Autodesk Fusion 360 part; units mm, degrees
(part 2 of 7)
  line L506 (63.504, -56.2361) -> (63.4239, -56.2507)
  line L507 (63.4239, -56.2507) -> (63.3435, -56.2671)
  line L508 (63.3435, -56.2671) -> (63.3141, -56.4047)
  line L509 (63.3141, -56.4047) -> (63.2867, -56.5426)
  line L510 (63.2867, -56.5426) -> (63.2612, -56.681)
  line L511 (63.2612, -56.681) -> (63.3292, -56.7269)
  line L512 (63.3292, -56.7269) -> (63.3976, -56.7711)
  line L513 (63.3976, -56.7711) -> (63.4664, -56.8134)
  line L514 (63.4664, -56.8134) -> (63.5357, -56.8539)
  line L515 (63.5357, -56.8539) -> (63.6053, -56.8924)
  line L516 (63.6053, -56.8924) -> (63.6754, -56.9288)
  line L517 (63.6754, -56.9288) -> (63.7458, -56.9631)
  line L518 (63.7458, -56.9631) -> (63.8167, -56.9949)
  line L519 (63.8167, -56.9949) -> (63.888, -57.0242)
  line L520 (63.888, -57.0242) -> (63.9598, -57.0505)
  line L521 (63.9598, -57.0505) -> (64.0322, -57.0732)
  line L522 (64.0322, -57.0732) -> (64.1053, -57.0906)
  line L523 (64.1053, -57.0906) -> (64.512, -57.1506)
  line L524 (64.512, -57.1506) -> (64.484, -57.3575)
  line L525 (64.484, -57.3575) -> (64.461, -57.565)
  line L526 (64.461, -57.565) -> (64.443, -57.7729)
  line L527 (64.443, -57.7729) -> (64.4301, -57.9813)
  line L528 (64.4301, -57.9813) -> (64.0196, -57.9609)
  line L529 (64.0196, -57.9609) -> (63.9445, -57.9636)
  line L530 (63.9445, -57.9636) -> (63.8691, -57.9718)
  line L531 (63.8691, -57.9718) -> (63.7935, -57.9836)
  line L532 (63.7935, -57.9836) -> (63.7179, -57.9984)
  line L533 (63.7179, -57.9984) -> (63.6421, -58.0158)
  line L534 (63.6421, -58.0158) -> (63.5664, -58.0356)
  line L535 (63.5664, -58.0356) -> (63.4905, -58.0577)
  line L536 (63.4905, -58.0577) -> (63.4147, -58.0818)
  line L537 (63.4147, -58.0818) -> (63.3389, -58.108)
  line L538 (63.3389, -58.108) -> (63.2632, -58.1361)
  line L539 (63.2632, -58.1361) -> (63.1874, -58.1661)
  line L540 (63.1874, -58.1661) -> (63.1118, -58.1979)
  line L541 (63.1118, -58.1979) -> (63.1098, -58.3386)
  line L542 (63.1098, -58.3386) -> (63.1098, -58.4792)
  line L543 (63.1098, -58.4792) -> (63.1118, -58.6199)
  line L544 (63.1118, -58.6199) -> (63.1874, -58.6517)
  line L545 (63.1874, -58.6517) -> (63.2632, -58.6817)
  line L546 (63.2632, -58.6817) -> (63.3389, -58.7098)
  line L547 (63.3389, -58.7098) -> (63.4147, -58.7359)
  line L548 (63.4147, -58.7359) -> (63.4905, -58.7601)
  line L549 (63.4905, -58.7601) -> (63.5664, -58.7822)
  line L550 (63.5664, -58.7822) -> (63.6421, -58.802)
  line L551 (63.6421, -58.802) -> (63.7179, -58.8194)
  line L552 (63.7179, -58.8194) -> (63.7935, -58.8342)
  line L553 (63.7935, -58.8342) -> (63.8691, -58.846)
  line L554 (63.8691, -58.846) -> (63.9445, -58.8542)
  line L555 (63.9445, -58.8542) -> (64.0196, -58.8569)
  line L556 (64.0196, -58.8569) -> (64.4301, -58.8365)
  line L557 (64.4301, -58.8365) -> (64.443, -59.0449)
  line L558 (64.443, -59.0449) -> (64.461, -59.2528)
  line L559 (64.461, -59.2528) -> (64.484, -59.4603)
  line L560 (64.484, -59.4603) -> (64.512, -59.6672)
  line L561 (64.512, -59.6672) -> (64.1053, -59.7272)
  line L562 (64.1053, -59.7272) -> (64.0322, -59.7446)
  line L563 (64.0322, -59.7446) -> (63.9598, -59.7673)
  line L564 (63.9598, -59.7673) -> (63.888, -59.7936)
  line L565 (63.888, -59.7936) -> (63.8167, -59.8229)
  line L566 (63.8167, -59.8229) -> (63.7458, -59.8547)
  line L567 (63.7458, -59.8547) -> (63.6754, -59.889)
  line L568 (63.6754, -59.889) -> (63.6053, -59.9254)
  line L569 (63.6053, -59.9254) -> (63.5357, -59.9639)
  line L570 (63.5357, -59.9639) -> (63.4664, -60.0044)
  line L571 (63.4664, -60.0044) -> (63.3976, -60.0467)
  line L572 (63.3976, -60.0467) -> (63.3292, -60.0909)
  line L573 (63.3292, -60.0909) -> (63.2612, -60.1368)
  line L574 (63.2612, -60.1368) -> (63.2867, -60.2752)
  line L575 (63.2867, -60.2752) -> (63.3141, -60.4131)
  line L576 (63.3141, -60.4131) -> (63.3435, -60.5507)
  line L577 (63.3435, -60.5507) -> (63.4239, -60.5671)
  line L578 (63.4239, -60.5671) -> (63.504, -60.5817)
  line L579 (63.504, -60.5817) -> (63.5838, -60.5945)
  line L580 (63.5838, -60.5945) -> (63.6633, -60.6054)
  line L581 (63.6633, -60.6054) -> (63.7424, -60.6143)
  line L582 (63.7424, -60.6143) -> (63.821, -60.6212)
  line L583 (63.821, -60.6212) -> (63.8992, -60.6258)
  line L584 (63.8992, -60.6258) -> (63.9769, -60.6282)
  line L585 (63.9769, -60.6282) -> (64.054, -60.6279)
  line L586 (64.054, -60.6279) -> (64.1304, -60.6247)
  line L587 (64.1304, -60.6247) -> (64.2059, -60.618)
  line L588 (64.2059, -60.618) -> (64.2801, -60.6061)
  line L589 (64.2801, -60.6061) -> (64.6788, -60.5059)
  line L590 (64.6788, -60.5059) -> (64.7321, -60.7078)
  line L591 (64.7321, -60.7078) -> (64.7903, -60.9083)
  line L592 (64.7903, -60.9083) -> (64.8533, -61.1073)
  line L593 (64.8533, -61.1073) -> (64.9211, -61.3047)
  line L594 (64.9211, -61.3047) -> (64.534, -61.4429)
  line L595 (64.534, -61.4429) -> (64.4656, -61.4742)
  line L596 (64.4656, -61.4742) -> (64.3991, -61.5106)
  line L597 (64.3991, -61.5106) -> (64.3338, -61.5504)
  line L598 (64.3338, -61.5504) -> (64.2696, -61.593)
  line L599 (64.2696, -61.593) -> (64.2063, -61.6381)
  line L600 (64.2063, -61.6381) -> (64.1438, -61.6854)
  line L601 (64.1438, -61.6854) -> (64.0823, -61.7348)
  line L602 (64.0823, -61.7348) -> (64.0215, -61.7862)
  line L603 (64.0215, -61.7862) -> (63.9614, -61.8394)
  line L604 (63.9614, -61.8394) -> (63.9022, -61.8943)
  line L605 (63.9022, -61.8943) -> (63.8437, -61.951)
  line L606 (63.8437, -61.951) -> (63.786, -62.0093)
  line L607 (63.786, -62.0093) -> (63.8379, -62.14)
  line L608 (63.8379, -62.14) -> (63.8918, -62.27)
  line L609 (63.8918, -62.27) -> (63.9475, -62.3992)
  line L610 (63.9475, -62.3992) -> (64.0295, -62.3996)
  line L611 (64.0295, -62.3996) -> (64.111, -62.3983)
  line L612 (64.111, -62.3983) -> (64.1917, -62.3953)
  line L613 (64.1917, -62.3953) -> (64.2718, -62.3905)
  line L614 (64.2718, -62.3905) -> (64.3511, -62.3838)
  line L615 (64.3511, -62.3838) -> (64.4295, -62.3752)
  line L616 (64.4295, -62.3752) -> (64.5071, -62.3645)
  line L617 (64.5071, -62.3645) -> (64.5838, -62.3516)
  line L618 (64.5838, -62.3516) -> (64.6593, -62.3363)
  line L619 (64.6593, -62.3363) -> (64.7336, -62.3183)
  line L620 (64.7336, -62.3183) -> (64.8064, -62.297)
  line L621 (64.8064, -62.297) -> (64.8769, -62.2708)
  line L622 (64.8769, -62.2708) -> (65.2484, -62.0948)
  line L623 (65.2484, -62.0948) -> (65.34, -62.2823)
  line L624 (65.34, -62.2823) -> (65.4362, -62.4676)
  line L625 (65.4362, -62.4676) -> (65.5368, -62.6505)
  line L626 (65.5368, -62.6505) -> (65.6418, -62.8309)
  line L627 (65.6418, -62.8309) -> (65.2891, -63.042)
  line L628 (65.2891, -63.042) -> (65.2282, -63.086)
  line L629 (65.2282, -63.086) -> (65.17, -63.1347)
  line L630 (65.17, -63.1347) -> (65.1138, -63.1865)
  line L631 (65.1138, -63.1865) -> (65.0591, -63.2408)
  line L632 (65.0591, -63.2408) -> (65.0058, -63.2974)
  line L633 (65.0058, -63.2974) -> (64.9538, -63.356)
  line L634 (64.9538, -63.356) -> (64.903, -63.4164)
  line L635 (64.903, -63.4164) -> (64.8534, -63.4787)
  line L636 (64.8534, -63.4787) -> (64.8049, -63.5425)
  line L637 (64.8049, -63.5425) -> (64.7575, -63.608)
  line L638 (64.7575, -63.608) -> (64.7112, -63.675)
  line L639 (64.7112, -63.675) -> (64.666, -63.7435)
  line L640 (64.666, -63.7435) -> (64.7425, -63.8615)
  line L641 (64.7425, -63.8615) -> (64.8206, -63.9785)
  line L642 (64.8206, -63.9785) -> (64.9004, -64.0943)
  line L643 (64.9004, -64.0943) -> (64.981, -64.0787)
  line L644 (64.981, -64.0787) -> (65.0606, -64.0616)
  line L645 (65.0606, -64.0616) -> (65.1392, -64.0429)
  line L646 (65.1392, -64.0429) -> (65.2168, -64.0225)
  line L647 (65.2168, -64.0225) -> (65.2933, -64.0005)
  line L648 (65.2933, -64.0005) -> (65.3686, -63.9767)
  line L649 (65.3686, -63.9767) -> (65.4426, -63.9511)
  line L650 (65.4426, -63.9511) -> (65.5152, -63.9235)
  line L651 (65.5152, -63.9235) -> (65.5864, -63.8938)
  line L652 (65.5864, -63.8938) -> (65.6557, -63.8616)
  line L653 (65.6557, -63.8616) -> (65.723, -63.8265)
  line L654 (65.723, -63.8265) -> (65.787, -63.7871)
  line L655 (65.787, -63.7871) -> (66.117, -63.542)
  line L656 (66.117, -63.542) -> (66.2434, -63.7081)
  line L657 (66.2434, -63.7081) -> (66.3739, -63.871)
  line L658 (66.3739, -63.871) -> (66.5083, -64.0308)
  line L659 (66.5083, -64.0308) -> (66.6465, -64.1872)
  line L660 (66.6465, -64.1872) -> (66.3418, -64.4631)
  line L661 (66.3418, -64.4631) -> (66.2906, -64.5181)
  line L662 (66.2906, -64.5181) -> (66.243, -64.5772)
  line L663 (66.243, -64.5772) -> (66.1979, -64.639)
  line L664 (66.1979, -64.639) -> (66.1549, -64.7029)
  line L665 (66.1549, -64.7029) -> (66.1137, -64.7688)
  line L666 (66.1137, -64.7688) -> (66.0741, -64.8364)
  line L667 (66.0741, -64.8364) -> (66.0361, -64.9056)
  line L668 (66.0361, -64.9056) -> (65.9996, -64.9763)
  line L669 (65.9996, -64.9763) -> (65.9645, -65.0484)
  line L670 (65.9645, -65.0484) -> (65.9308, -65.1219)
  line L671 (65.9308, -65.1219) -> (65.8984, -65.1966)
  line L672 (65.8984, -65.1966) -> (65.8674, -65.2726)
  line L673 (65.8674, -65.2726) -> (65.9655, -65.3735)
  line L674 (65.9655, -65.3735) -> (66.0649, -65.473)
  line L675 (66.0649, -65.473) -> (66.1658, -65.571)
  line L676 (66.1658, -65.571) -> (66.2418, -65.54)
  line L677 (66.2418, -65.54) -> (66.3165, -65.5076)
  line L678 (66.3165, -65.5076) -> (66.39, -65.4739)
  line L679 (66.39, -65.4739) -> (66.4621, -65.4388)
  line L680 (66.4621, -65.4388) -> (66.5328, -65.4023)
  line L681 (66.5328, -65.4023) -> (66.602, -65.3643)
  line L682 (66.602, -65.3643) -> (66.6696, -65.3248)
  line L683 (66.6696, -65.3248) -> (66.7355, -65.2835)
  line L684 (66.7355, -65.2835) -> (66.7994, -65.2405)
  line L685 (66.7994, -65.2405) -> (66.8612, -65.1954)
  line L686 (66.8612, -65.1954) -> (66.9203, -65.1479)
  line L687 (66.9203, -65.1479) -> (66.9753, -65.0967)
  line L688 (66.9753, -65.0967) -> (67.2512, -64.7919)
  line L689 (67.2512, -64.7919) -> (67.4076, -64.9301)
  line L690 (67.4076, -64.9301) -> (67.5674, -65.0645)
  line L691 (67.5674, -65.0645) -> (67.7304, -65.195)
  line L692 (67.7304, -65.195) -> (67.8964, -65.3215)
  line L693 (67.8964, -65.3215) -> (67.6514, -65.6515)
  line L694 (67.6514, -65.6515) -> (67.6119, -65.7155)
  line L695 (67.6119, -65.7155) -> (67.5768, -65.7827)
  line L696 (67.5768, -65.7827) -> (67.5446, -65.8521)
  line L697 (67.5446, -65.8521) -> (67.5149, -65.9232)
  line L698 (67.5149, -65.9232) -> (67.4873, -65.9958)
  line L699 (67.4873, -65.9958) -> (67.4617, -66.0698)
  line L700 (67.4617, -66.0698) -> (67.4379, -66.1451)
  line L701 (67.4379, -66.1451) -> (67.4159, -66.2216)
  line L702 (67.4159, -66.2216) -> (67.3956, -66.2992)
  line L703 (67.3956, -66.2992) -> (67.3768, -66.3778)
  line L704 (67.3768, -66.3778) -> (67.3597, -66.4574)
  line L705 (67.3597, -66.4574) -> (67.3441, -66.538)
  line L706 (67.3441, -66.538) -> (67.4599, -66.6178)
  line L707 (67.4599, -66.6178) -> (67.5769, -66.6959)
  line L708 (67.5769, -66.6959) -> (67.695, -66.7724)
  line L709 (67.695, -66.7724) -> (67.7634, -66.7272)
  line L710 (67.7634, -66.7272) -> (67.8304, -66.6809)
  line L711 (67.8304, -66.6809) -> (67.8959, -66.6335)
  line L712 (67.8959, -66.6335) -> (67.9598, -66.585)
  line L713 (67.9598, -66.585) -> (68.022, -66.5354)
  line L714 (68.022, -66.5354) -> (68.0824, -66.4846)
  line L715 (68.0824, -66.4846) -> (68.141, -66.4326)
  line L716 (68.141, -66.4326) -> (68.1976, -66.3793)
  line L717 (68.1976, -66.3793) -> (68.2519, -66.3246)
  line L718 (68.2519, -66.3246) -> (68.3037, -66.2684)
  line L719 (68.3037, -66.2684) -> (68.3524, -66.2102)
  line L720 (68.3524, -66.2102) -> (68.3964, -66.1493)
  line L721 (68.3964, -66.1493) -> (68.6075, -65.7966)
  line L722 (68.6075, -65.7966) -> (68.7879, -65.9016)
  line L723 (68.7879, -65.9016) -> (68.9708, -66.0022)
  line L724 (68.9708, -66.0022) -> (69.1561, -66.0984)
  line L725 (69.1561, -66.0984) -> (69.3436, -66.19)
  line L726 (69.3436, -66.19) -> (69.1677, -66.5615)
  line L727 (69.1677, -66.5615) -> (69.1414, -66.632)
  line L728 (69.1414, -66.632) -> (69.1201, -66.7048)
  line L729 (69.1201, -66.7048) -> (69.1021, -66.7791)
  line L730 (69.1021, -66.7791) -> (69.0868, -66.8546)
  line L731 (69.0868, -66.8546) -> (69.0739, -66.9313)
  line L732 (69.0739, -66.9313) -> (69.0633, -67.0089)
  line L733 (69.0633, -67.0089) -> (69.0546, -67.0874)
  line L734 (69.0546, -67.0874) -> (69.0479, -67.1666)
  line L735 (69.0479, -67.1666) -> (69.0431, -67.2467)
  line L736 (69.0431, -67.2467) -> (69.0401, -67.3275)
  line L737 (69.0401, -67.3275) -> (69.0388, -67.4089)
  line L738 (69.0388, -67.4089) -> (69.0392, -67.491)
  line L739 (69.0392, -67.491) -> (69.1684, -67.5466)
  line L740 (69.1684, -67.5466) -> (69.2984, -67.6005)
  line L741 (69.2984, -67.6005) -> (69.4291, -67.6525)
  line L742 (69.4291, -67.6525) -> (69.4874, -67.5947)
  line L743 (69.4874, -67.5947) -> (69.5441, -67.5362)
  line L744 (69.5441, -67.5362) -> (69.5991, -67.477)
  line L745 (69.5991, -67.477) -> (69.6523, -67.417)
  line L746 (69.6523, -67.417) -> (69.7036, -67.3562)
  line L747 (69.7036, -67.3562) -> (69.753, -67.2946)
  line L748 (69.753, -67.2946) -> (69.8003, -67.2321)
  line L749 (69.8003, -67.2321) -> (69.8454, -67.1689)
  line L750 (69.8454, -67.1689) -> (69.888, -67.1046)
  line L751 (69.888, -67.1046) -> (69.9278, -67.0393)
  line L752 (69.9278, -67.0393) -> (69.9642, -66.9728)
  line L753 (69.9642, -66.9728) -> (69.9955, -66.9044)
  line L754 (69.9955, -66.9044) -> (70.1337, -66.5173)
  line L755 (70.1337, -66.5173) -> (70.3312, -66.5851)
  line L756 (70.3312, -66.5851) -> (70.5302, -66.6482)
  line L757 (70.5302, -66.6482) -> (70.7306, -66.7063)
  line L758 (70.7306, -66.7063) -> (70.9325, -66.7596)
  line L759 (70.9325, -66.7596) -> (70.8324, -67.1583)
  line L760 (70.8324, -67.1583) -> (70.8204, -67.2325)
  line L761 (70.8204, -67.2325) -> (70.8137, -67.3081)
  line L762 (70.8137, -67.3081) -> (70.8105, -67.3845)
  line L763 (70.8105, -67.3845) -> (70.8103, -67.4615)
  line L764 (70.8103, -67.4615) -> (70.8126, -67.5392)
  line L765 (70.8126, -67.5392) -> (70.8172, -67.6174)
  line L766 (70.8172, -67.6174) -> (70.8241, -67.6961)
  line L767 (70.8241, -67.6961) -> (70.833, -67.7751)
  line L768 (70.833, -67.7751) -> (70.8439, -67.8546)
  line L769 (70.8439, -67.8546) -> (70.8567, -67.9344)
  line L770 (70.8567, -67.9344) -> (70.8713, -68.0145)
  line L771 (70.8713, -68.0145) -> (70.8877, -68.0949)
  line L772 (70.8877, -68.0949) -> (71.0253, -68.1243)
  line L773 (71.0253, -68.1243) -> (71.1633, -68.1518)
  line L774 (71.1633, -68.1518) -> (71.3016, -68.1773)
  line L775 (71.3016, -68.1773) -> (71.3475, -68.1092)
  line L776 (71.3475, -68.1092) -> (71.3917, -68.0408)
  line L777 (71.3917, -68.0408) -> (71.4341, -67.972)
  line L778 (71.4341, -67.972) -> (71.4745, -67.9027)
  line L779 (71.4745, -67.9027) -> (71.513, -67.8331)
  line L780 (71.513, -67.8331) -> (71.5495, -67.7631)
  line L781 (71.5495, -67.7631) -> (71.5837, -67.6926)
  line L782 (71.5837, -67.6926) -> (71.6156, -67.6217)
  line L783 (71.6156, -67.6217) -> (71.6448, -67.5504)
  line L784 (71.6448, -67.5504) -> (71.6711, -67.4786)
  line L785 (71.6711, -67.4786) -> (71.6938, -67.4063)
  line L786 (71.6938, -67.4063) -> (71.7112, -67.3331)
  line L787 (71.7112, -67.3331) -> (71.7713, -66.9265)
  line L788 (71.7713, -66.9265) -> (71.9781, -66.9545)
  line L789 (71.9781, -66.9545) -> (72.1856, -66.9774)
  line L790 (72.1856, -66.9774) -> (72.3936, -66.9954)
  line L791 (72.3936, -66.9954) -> (72.6019, -67.0083)
  line L792 (72.6019, -67.0083) -> (72.5815, -67.4188)
  line L793 (72.5815, -67.4188) -> (72.5842, -67.494)
  line L794 (72.5842, -67.494) -> (72.5924, -67.5694)
  line L795 (72.5924, -67.5694) -> (72.6042, -67.6449)
  line L796 (72.6042, -67.6449) -> (72.619, -67.7206)
  line L797 (72.619, -67.7206) -> (72.6364, -67.7963)
  line L798 (72.6364, -67.7963) -> (72.6562, -67.8721)
  line L799 (72.6562, -67.8721) -> (72.6783, -67.9479)
  line L800 (72.6783, -67.9479) -> (72.7025, -68.0237)
  line L801 (72.7025, -68.0237) -> (72.7287, -68.0995)
  line L802 (72.7287, -68.0995) -> (72.7568, -68.1753)
  line L803 (72.7568, -68.1753) -> (72.7867, -68.251)
  line L804 (72.7867, -68.251) -> (72.8185, -68.3267)
  line L805 (72.8185, -68.3267) -> (72.9592, -68.3286)
  line L806 (72.9592, -68.3286) -> (73.0999, -68.3286)
  line L807 (73.0999, -68.3286) -> (73.2405, -68.3267)
  line L808 (73.2405, -68.3267) -> (73.2723, -68.251)
  line L809 (73.2723, -68.251) -> (73.3023, -68.1753)
  line L810 (73.3023, -68.1753) -> (73.3304, -68.0995)
  line L811 (73.3304, -68.0995) -> (73.3566, -68.0237)
  line L812 (73.3566, -68.0237) -> (73.3807, -67.9479)
  line L813 (73.3807, -67.9479) -> (73.4028, -67.8721)
  line L814 (73.4028, -67.8721) -> (73.4226, -67.7963)
  line L815 (73.4226, -67.7963) -> (73.4401, -67.7206)
  line L816 (73.4401, -67.7206) -> (73.4548, -67.6449)
  line L817 (73.4548, -67.6449) -> (73.4666, -67.5694)
  line L818 (73.4666, -67.5694) -> (73.4748, -67.494)
  line L819 (73.4748, -67.494) -> (73.4775, -67.4188)
  line L820 (73.4775, -67.4188) -> (73.4571, -67.0083)
  line L821 (73.4571, -67.0083) -> (73.6655, -66.9954)
  line L822 (73.6655, -66.9954) -> (73.8734, -66.9774)
  line L823 (73.8734, -66.9774) -> (74.0809, -66.9545)
  line L824 (74.0809, -66.9545) -> (74.2878, -66.9265)
  line L825 (74.2878, -66.9265) -> (74.3479, -67.3331)
  line L826 (74.3479, -67.3331) -> (74.3652, -67.4063)
  line L827 (74.3652, -67.4063) -> (74.3879, -67.4786)
  line L828 (74.3879, -67.4786) -> (74.4142, -67.5504)
  line L829 (74.4142, -67.5504) -> (74.4435, -67.6217)
  line L830 (74.4435, -67.6217) -> (74.4753, -67.6926)
  line L831 (74.4753, -67.6926) -> (74.5096, -67.7631)
  line L832 (74.5096, -67.7631) -> (74.546, -67.8331)
  line L833 (74.546, -67.8331) -> (74.5845, -67.9027)
  line L834 (74.5845, -67.9027) -> (74.625, -67.972)
  line L835 (74.625, -67.972) -> (74.6673, -68.0408)
  line L836 (74.6673, -68.0408) -> (74.7115, -68.1092)
  line L837 (74.7115, -68.1092) -> (74.7574, -68.1773)
  line L838 (74.7574, -68.1773) -> (74.8958, -68.1518)
  line L839 (74.8958, -68.1518) -> (75.0338, -68.1243)
  line L840 (75.0338, -68.1243) -> (75.1713, -68.0949)
  line L841 (75.1713, -68.0949) -> (75.1877, -68.0145)
  line L842 (75.1877, -68.0145) -> (75.2024, -67.9344)
  line L843 (75.2024, -67.9344) -> (75.2151, -67.8546)
  line L844 (75.2151, -67.8546) -> (75.226, -67.7751)
  line L845 (75.226, -67.7751) -> (75.235, -67.6961)
  line L846 (75.235, -67.6961) -> (75.2418, -67.6174)
  line L847 (75.2418, -67.6174) -> (75.2465, -67.5392)
  line L848 (75.2465, -67.5392) -> (75.2488, -67.4615)
  line L849 (75.2488, -67.4615) -> (75.2485, -67.3845)
  line L850 (75.2485, -67.3845) -> (75.2453, -67.3081)
  line L851 (75.2453, -67.3081) -> (75.2387, -67.2325)
  line L852 (75.2387, -67.2325) -> (75.2267, -67.1583)
  line L853 (75.2267, -67.1583) -> (75.1266, -66.7596)
  line L854 (75.1266, -66.7596) -> (75.3284, -66.7063)
  line L855 (75.3284, -66.7063) -> (75.5289, -66.6482)
  line L856 (75.5289, -66.6482) -> (75.7279, -66.5851)
  line L857 (75.7279, -66.5851) -> (75.9253, -66.5173)
  line L858 (75.9253, -66.5173) -> (76.0636, -66.9044)
  line L859 (76.0636, -66.9044) -> (76.0948, -66.9728)
  line L860 (76.0948, -66.9728) -> (76.1312, -67.0393)
  line L861 (76.1312, -67.0393) -> (76.171, -67.1046)
  line L862 (76.171, -67.1046) -> (76.2137, -67.1689)
  line L863 (76.2137, -67.1689) -> (76.2587, -67.2321)
  line L864 (76.2587, -67.2321) -> (76.306, -67.2946)
  line L865 (76.306, -67.2946) -> (76.3554, -67.3562)
  line L866 (76.3554, -67.3562) -> (76.4068, -67.417)
  line L867 (76.4068, -67.417) -> (76.46, -67.477)
  line L868 (76.46, -67.477) -> (76.515, -67.5362)
  line L869 (76.515, -67.5362) -> (76.5716, -67.5947)
  line L870 (76.5716, -67.5947) -> (76.6299, -67.6525)
  line L871 (76.6299, -67.6525) -> (76.7607, -67.6005)
  line L872 (76.7607, -67.6005) -> (76.8906, -67.5466)
  line L873 (76.8906, -67.5466) -> (77.0198, -67.491)
  line L874 (77.0198, -67.491) -> (77.0202, -67.4089)
  line L875 (77.0202, -67.4089) -> (77.0189, -67.3275)
  line L876 (77.0189, -67.3275) -> (77.0159, -67.2467)
  line L877 (77.0159, -67.2467) -> (77.0111, -67.1666)
  line L878 (77.0111, -67.1666) -> (77.0044, -67.0874)
  line L879 (77.0044, -67.0874) -> (76.9958, -67.0089)
  line L880 (76.9958, -67.0089) -> (76.9851, -66.9313)
  line L881 (76.9851, -66.9313) -> (76.9722, -66.8546)
  line L882 (76.9722, -66.8546) -> (76.9569, -66.7791)
  line L883 (76.9569, -66.7791) -> (76.9389, -66.7048)
  line L884 (76.9389, -66.7048) -> (76.9176, -66.632)
  line L885 (76.9176, -66.632) -> (76.8914, -66.5615)
  line L886 (76.8914, -66.5615) -> (76.7154, -66.19)
  line L887 (76.7154, -66.19) -> (76.903, -66.0984)
  line L888 (76.903, -66.0984) -> (77.0882, -66.0022)
  line L889 (77.0882, -66.0022) -> (77.2711, -65.9016)
  line L890 (77.2711, -65.9016) -> (77.4515, -65.7966)
  line L891 (77.4515, -65.7966) -> (77.6626, -66.1493)
  line L892 (77.6626, -66.1493) -> (77.7067, -66.2102)
  line L893 (77.7067, -66.2102) -> (77.7553, -66.2684)
  line L894 (77.7553, -66.2684) -> (77.8071, -66.3246)
  line L895 (77.8071, -66.3246) -> (77.8615, -66.3793)
  line L896 (77.8615, -66.3793) -> (77.918, -66.4326)
  line L897 (77.918, -66.4326) -> (77.9766, -66.4846)
  line L898 (77.9766, -66.4846) -> (78.0371, -66.5354)
  line L899 (78.0371, -66.5354) -> (78.0993, -66.585)
  line L900 (78.0993, -66.585) -> (78.1632, -66.6335)
  line L901 (78.1632, -66.6335) -> (78.2286, -66.6809)
  line L902 (78.2286, -66.6809) -> (78.2956, -66.7272)
  line L903 (78.2956, -66.7272) -> (78.3641, -66.7724)
  line L904 (78.3641, -66.7724) -> (78.4822, -66.6959)
  line L905 (78.4822, -66.6959) -> (78.5991, -66.6178)
  line L906 (78.5991, -66.6178) -> (78.715, -66.538)
  line L907 (78.715, -66.538) -> (78.6994, -66.4574)
  line L908 (78.6994, -66.4574) -> (78.6822, -66.3778)
  line L909 (78.6822, -66.3778) -> (78.6635, -66.2992)
  line L910 (78.6635, -66.2992) -> (78.6431, -66.2216)
  line L911 (78.6431, -66.2216) -> (78.6211, -66.1451)
  line L912 (78.6211, -66.1451) -> (78.5974, -66.0698)
  line L913 (78.5974, -66.0698) -> (78.5717, -65.9958)
  line L914 (78.5717, -65.9958) -> (78.5441, -65.9232)
  line L915 (78.5441, -65.9232) -> (78.5144, -65.8521)
  line L916 (78.5144, -65.8521) -> (78.4822, -65.7827)
  line L917 (78.4822, -65.7827) -> (78.4471, -65.7155)
  line L918 (78.4471, -65.7155) -> (78.4077, -65.6515)
  line L919 (78.4077, -65.6515) -> (78.1626, -65.3215)
  line L920 (78.1626, -65.3215) -> (78.3287, -65.195)
  line L921 (78.3287, -65.195) -> (78.4916, -65.0645)
  line L922 (78.4916, -65.0645) -> (78.6514, -64.9301)
  line L923 (78.6514, -64.9301) -> (78.8078, -64.7919)
  line L924 (78.8078, -64.7919) -> (79.0837, -65.0967)
  line L925 (79.0837, -65.0967) -> (79.1388, -65.1479)
  line L926 (79.1388, -65.1479) -> (79.1979, -65.1954)
  line L927 (79.1979, -65.1954) -> (79.2596, -65.2405)
  line L928 (79.2596, -65.2405) -> (79.3236, -65.2835)
  line L929 (79.3236, -65.2835) -> (79.3894, -65.3248)
  line L930 (79.3894, -65.3248) -> (79.457, -65.3643)
  line L931 (79.457, -65.3643) -> (79.5262, -65.4023)
  line L932 (79.5262, -65.4023) -> (79.5969, -65.4388)
  line L933 (79.5969, -65.4388) -> (79.6691, -65.4739)
  line L934 (79.6691, -65.4739) -> (79.7425, -65.5076)
  line L935 (79.7425, -65.5076) -> (79.8173, -65.54)
  line L936 (79.8173, -65.54) -> (79.8932, -65.571)
  line L937 (79.8932, -65.571) -> (79.9941, -65.473)
  line L938 (79.9941, -65.473) -> (80.0936, -65.3735)
  line L939 (80.0936, -65.3735) -> (80.1916, -65.2726)
  line L940 (80.1916, -65.2726) -> (80.1606, -65.1966)
  line L941 (80.1606, -65.1966) -> (80.1283, -65.1219)
  line L942 (80.1283, -65.1219) -> (80.0945, -65.0484)
  line L943 (80.0945, -65.0484) -> (80.0595, -64.9763)
  line L944 (80.0595, -64.9763) -> (80.0229, -64.9056)
  line L945 (80.0229, -64.9056) -> (79.9849, -64.8364)
  line L946 (79.9849, -64.8364) -> (79.9454, -64.7688)
  line L947 (79.9454, -64.7688) -> (79.9041, -64.7029)
  line L948 (79.9041, -64.7029) -> (79.8611, -64.639)
  line L949 (79.8611, -64.639) -> (79.816, -64.5772)
  line L950 (79.816, -64.5772) -> (79.7685, -64.5181)
  line L951 (79.7685, -64.5181) -> (79.7173, -64.4631)
  line L952 (79.7173, -64.4631) -> (79.4126, -64.1872)
  line L953 (79.4126, -64.1872) -> (79.5508, -64.0308)
  line L954 (79.5508, -64.0308) -> (79.6851, -63.871)
  line L955 (79.6851, -63.871) -> (79.8156, -63.7081)
  line L956 (79.8156, -63.7081) -> (79.9421, -63.542)
  line L957 (79.9421, -63.542) -> (80.2721, -63.7871)
  line L958 (80.2721, -63.7871) -> (80.3361, -63.8265)
  line L959 (80.3361, -63.8265) -> (80.4033, -63.8616)
  line L960 (80.4033, -63.8616) -> (80.4727, -63.8938)
  line L961 (80.4727, -63.8938) -> (80.5438, -63.9235)
  line L962 (80.5438, -63.9235) -> (80.6164, -63.9511)
  line L963 (80.6164, -63.9511) -> (80.6905, -63.9767)
  line L964 (80.6905, -63.9767) -> (80.7658, -64.0005)
  line L965 (80.7658, -64.0005) -> (80.8422, -64.0225)
  line L966 (80.8422, -64.0225) -> (80.9198, -64.0429)
  line L967 (80.9198, -64.0429) -> (80.9984, -64.0616)
  line L968 (80.9984, -64.0616) -> (81.078, -64.0787)
  line L969 (81.078, -64.0787) -> (81.1586, -64.0943)
  line L970 (81.1586, -64.0943) -> (81.2384, -63.9785)
  line L971 (81.2384, -63.9785) -> (81.3166, -63.8615)
  line L972 (81.3166, -63.8615) -> (81.3931, -63.7435)
  line L973 (81.3931, -63.7435) -> (81.3478, -63.675)
  line L974 (81.3478, -63.675) -> (81.3015, -63.608)
  line L975 (81.3015, -63.608) -> (81.2541, -63.5425)
  line L976 (81.2541, -63.5425) -> (81.2056, -63.4787)
  line L977 (81.2056, -63.4787) -> (81.156, -63.4164)
  line L978 (81.156, -63.4164) -> (81.1052, -63.356)
  line L979 (81.1052, -63.356) -> (81.0532, -63.2974)
  line L980 (81.0532, -63.2974) -> (81, -63.2408)
  line L981 (81, -63.2408) -> (80.9453, -63.1865)
  line L982 (80.9453, -63.1865) -> (80.889, -63.1347)
  line L983 (80.889, -63.1347) -> (80.8309, -63.086)
  line L984 (80.8309, -63.086) -> (80.7699, -63.042)
  line L985 (80.7699, -63.042) -> (80.4172, -62.8309)
  line L986 (80.4172, -62.8309) -> (80.5222, -62.6505)
  line L987 (80.5222, -62.6505) -> (80.6229, -62.4676)
  line L988 (80.6229, -62.4676) -> (80.719, -62.2823)
  line L989 (80.719, -62.2823) -> (80.8107, -62.0948)
  line L990 (80.8107, -62.0948) -> (81.1821, -62.2708)
  line L991 (81.1821, -62.2708) -> (81.2526, -62.297)
  line L992 (81.2526, -62.297) -> (81.3254, -62.3183)
  line L993 (81.3254, -62.3183) -> (81.3997, -62.3363)
  line L994 (81.3997, -62.3363) -> (81.4753, -62.3516)
  line L995 (81.4753, -62.3516) -> (81.5519, -62.3645)
  line L996 (81.5519, -62.3645) -> (81.6295, -62.3752)
  line L997 (81.6295, -62.3752) -> (81.708, -62.3838)
  line L998 (81.708, -62.3838) -> (81.7873, -62.3905)
  line L999 (81.7873, -62.3905) -> (81.8673, -62.3953)
  line L1000 (81.8673, -62.3953) -> (81.9481, -62.3983)
  line L1001 (81.9481, -62.3983) -> (82.0295, -62.3996)
  line L1002 (82.0295, -62.3996) -> (82.1116, -62.3992)
  line L1003 (82.1116, -62.3992) -> (82.1673, -62.27)
  line L1004 (82.1673, -62.27) -> (82.2211, -62.14)
  line L1005 (82.2211, -62.14) -> (82.2731, -62.0093)
  line L1006 (82.2731, -62.0093) -> (82.2153, -61.951)
  line L1007 (82.2153, -61.951) -> (82.1568, -61.8943)
  line L1008 (82.1568, -61.8943) -> (82.0976, -61.8394)
  line L1009 (82.0976, -61.8394) -> (82.0376, -61.7862)
  line L1010 (82.0376, -61.7862) -> (81.9768, -61.7348)
  line L1011 (81.9768, -61.7348) -> (81.9152, -61.6854)
  line L1012 (81.9152, -61.6854) -> (81.8528, -61.6381)
  line L1013 (81.8528, -61.6381) -> (81.7895, -61.593)
  line L1014 (81.7895, -61.593) -> (81.7252, -61.5504)
  line L1015 (81.7252, -61.5504) -> (81.6599, -61.5106)
  line L1016 (81.6599, -61.5106) -> (81.5934, -61.4742)
  line L1017 (81.5934, -61.4742) -> (81.525, -61.4429)
  line L1018 (81.525, -61.4429) -> (81.1379, -61.3047)
  line L1019 (81.1379, -61.3047) -> (81.2058, -61.1073)
  line L1020 (81.2058, -61.1073) -> (81.2688, -60.9083)
  line L1021 (81.2688, -60.9083) -> (81.3269, -60.7078)
  line L1022 (81.3269, -60.7078) -> (81.3802, -60.5059)
  line L1023 (81.3802, -60.5059) -> (81.7789, -60.6061)
  line L1024 (81.7789, -60.6061) -> (81.8531, -60.618)
  line L1025 (81.8531, -60.618) -> (81.9287, -60.6247)
  line L1026 (81.9287, -60.6247) -> (82.0051, -60.6279)
  line L1027 (82.0051, -60.6279) -> (82.0822, -60.6282)
  line L1028 (82.0822, -60.6282) -> (82.1598, -60.6258)
  line L1029 (82.1598, -60.6258) -> (82.238, -60.6212)
  line L1030 (82.238, -60.6212) -> (82.3167, -60.6143)
  line L1031 (82.3167, -60.6143) -> (82.3958, -60.6054)
  line L1032 (82.3958, -60.6054) -> (82.4752, -60.5945)
  line L1033 (82.4752, -60.5945) -> (82.555, -60.5817)
  line L1034 (82.555, -60.5817) -> (82.6351, -60.5671)
  line L1035 (82.6351, -60.5671) -> (82.7155, -60.5507)
  line L1036 (82.7155, -60.5507) -> (82.7449, -60.4131)
  line L1037 (82.7449, -60.4131) -> (82.7724, -60.2752)
  line L1038 (82.7724, -60.2752) -> (82.7979, -60.1368)
  line L1039 (82.7979, -60.1368) -> (82.7299, -60.0909)
  line L1040 (82.7299, -60.0909) -> (82.6614, -60.0467)
  line L1041 (82.6614, -60.0467) -> (82.5926, -60.0044)
  line L1042 (82.5926, -60.0044) -> (82.5234, -59.9639)
  line L1043 (82.5234, -59.9639) -> (82.4537, -59.9254)
  line L1044 (82.4537, -59.9254) -> (82.3837, -59.889)
  line L1045 (82.3837, -59.889) -> (82.3132, -59.8547)
  line L1046 (82.3132, -59.8547) -> (82.2423, -59.8229)
  line L1047 (82.2423, -59.8229) -> (82.171, -59.7936)
  line L1048 (82.171, -59.7936) -> (82.0992, -59.7673)
  line L1049 (82.0992, -59.7673) -> (82.0269, -59.7446)
  line L1050 (82.0269, -59.7446) -> (81.9537, -59.7272)
  line L1051 (81.9537, -59.7272) -> (81.5471, -59.6672)
  line L1052 (81.5471, -59.6672) -> (81.5751, -59.4603)
  line L1053 (81.5751, -59.4603) -> (81.5981, -59.2528)
  line L1054 (81.5981, -59.2528) -> (81.616, -59.0449)
  line L1055 (81.616, -59.0449) -> (81.6289, -58.8365)
  circle A0 centre (73.0295, -58.4089) radius 2.2
extrude "Extrude1'" add sketch "Sketch1 (2)" along normal blind 2 separate body makes body 2 in component "CT idler 1"
ref_plane "WorkPlane2" through (0, 0, 39) normal (0, 0, 1) x (1, 0, 0) in component "CT idler 1"
sketch "Sketch2" plane through (0, 0, 39) normal (0, 0, 1) x (1, 0, 0) in component "CT idler 1"
  line L0 (76.0819, -58.8895) -> (76.3712, -58.9351)
  line L1 (76.3712, -58.9351) -> (76.4518, -58.9359)
  line L2 (76.4518, -58.9359) -> (76.5339, -58.9268)
  line L3 (76.5339, -58.9268) -> (76.6168, -58.9107)
  line L4 (76.6168, -58.9107) -> (76.7002, -58.8887)
  line L5 (76.7002, -58.8887) -> (76.7841, -58.8612)
  line L6 (76.7841, -58.8612) -> (76.8681, -58.8287)
  line L7 (76.8681, -58.8287) -> (76.9521, -58.7913)
  line L8 (76.9521, -58.7913) -> (77.036, -58.7493)
  line L9 (77.036, -58.7493) -> (77.1197, -58.7028)
  line L10 (77.1197, -58.7028) -> (77.2029, -58.6518)
  line L11 (77.2029, -58.6518) -> (77.2856, -58.5964)
  line L12 (77.2856, -58.5964) -> (77.3676, -58.5368)
  line L13 (77.3676, -58.5368) -> (77.3693, -58.4515)
  line L14 (77.3693, -58.4515) -> (77.3693, -58.3662)
  line L15 (77.3693, -58.3662) -> (77.3676, -58.281)
  line L16 (77.3676, -58.281) -> (77.2856, -58.2214)
  line L17 (77.2856, -58.2214) -> (77.2029, -58.166)
  line L18 (77.2029, -58.166) -> (77.1197, -58.115)
  line L19 (77.1197, -58.115) -> (77.036, -58.0685)
  line L20 (77.036, -58.0685) -> (76.9521, -58.0265)
  line L21 (76.9521, -58.0265) -> (76.8681, -57.9891)
  line L22 (76.8681, -57.9891) -> (76.7841, -57.9566)
  line L23 (76.7841, -57.9566) -> (76.7002, -57.9291)
  line L24 (76.7002, -57.9291) -> (76.6168, -57.9071)
  line L25 (76.6168, -57.9071) -> (76.5339, -57.891)
  line L26 (76.5339, -57.891) -> (76.4518, -57.8819)
  line L27 (76.4518, -57.8819) -> (76.3712, -57.8827)
  line L28 (76.3712, -57.8827) -> (76.0819, -57.9283)
  line L29 (76.0819, -57.9283) -> (76.0523, -57.7678)
  line L30 (76.0523, -57.7678) -> (76.0142, -57.6091)
  line L31 (76.0142, -57.6091) -> (75.9679, -57.4527)
  line L32 (75.9679, -57.4527) -> (75.9133, -57.2989)
  line L33 (75.9133, -57.2989) -> (76.1866, -57.1937)
  line L34 (76.1866, -57.1937) -> (76.2568, -57.1542)
  line L35 (76.2568, -57.1542) -> (76.3233, -57.1052)
  line L36 (76.3233, -57.1052) -> (76.3871, -57.0499)
  line L37 (76.3871, -57.0499) -> (76.4483, -56.989)
  line L38 (76.4483, -56.989) -> (76.5072, -56.9233)
  line L39 (76.5072, -56.9233) -> (76.5637, -56.8532)
  line L40 (76.5637, -56.8532) -> (76.6178, -56.7788)
  line L41 (76.6178, -56.7788) -> (76.6695, -56.7005)
  line L42 (76.6695, -56.7005) -> (76.7187, -56.6183)
  line L43 (76.7187, -56.6183) -> (76.7652, -56.5325)
  line L44 (76.7652, -56.5325) -> (76.8092, -56.4433)
  line L45 (76.8092, -56.4433) -> (76.8504, -56.3506)
  line L46 (76.8504, -56.3506) -> (76.8092, -56.2759)
  line L47 (76.8092, -56.2759) -> (76.7666, -56.2021)
  line L48 (76.7666, -56.2021) -> (76.7225, -56.129)
  line L49 (76.7225, -56.129) -> (76.6217, -56.1184)
  line L50 (76.6217, -56.1184) -> (76.5224, -56.1119)
  line L51 (76.5224, -56.1119) -> (76.4248, -56.1093)
  line L52 (76.4248, -56.1093) -> (76.3291, -56.1108)
  line L53 (76.3291, -56.1108) -> (76.2354, -56.1164)
  line L54 (76.2354, -56.1164) -> (76.1439, -56.1261)
  line L55 (76.1439, -56.1261) -> (76.0549, -56.1399)
  line L56 (76.0549, -56.1399) -> (75.9686, -56.1581)
  line L57 (75.9686, -56.1581) -> (75.8853, -56.1807)
  line L58 (75.8853, -56.1807) -> (75.8054, -56.2082)
  line L59 (75.8054, -56.2082) -> (75.7298, -56.2413)
  line L60 (75.7298, -56.2413) -> (75.6604, -56.2823)
  line L61 (75.6604, -56.2823) -> (75.4327, -56.4665)
  line L62 (75.4327, -56.4665) -> (75.3268, -56.3423)
  line L63 (75.3268, -56.3423) -> (75.2145, -56.2239)
  line L64 (75.2145, -56.2239) -> (75.0961, -56.1117)
  line L65 (75.0961, -56.1117) -> (74.972, -56.0058)
  line L66 (74.972, -56.0058) -> (75.1561, -55.778)
  line L67 (75.1561, -55.778) -> (75.1971, -55.7086)
  line L68 (75.1971, -55.7086) -> (75.2302, -55.633)
  line L69 (75.2302, -55.633) -> (75.2577, -55.5532)
  line L70 (75.2577, -55.5532) -> (75.2804, -55.4699)
  line L71 (75.2804, -55.4699) -> (75.2985, -55.3835)
  line L72 (75.2985, -55.3835) -> (75.3124, -55.2945)
  line L73 (75.3124, -55.2945) -> (75.322, -55.203)
  line L74 (75.322, -55.203) -> (75.3276, -55.1094)
  line L75 (75.3276, -55.1094) -> (75.3291, -55.0136)
  line L76 (75.3291, -55.0136) -> (75.3266, -54.916)
  line L77 (75.3266, -54.916) -> (75.32, -54.8168)
  line L78 (75.32, -54.8168) -> (75.3094, -54.7159)
  line L79 (75.3094, -54.7159) -> (75.2364, -54.6719)
  line L80 (75.2364, -54.6719) -> (75.1625, -54.6292)
  line L81 (75.1625, -54.6292) -> (75.0878, -54.588)
  line L82 (75.0878, -54.588) -> (74.9952, -54.6292)
  line L83 (74.9952, -54.6292) -> (74.9059, -54.6732)
  line L84 (74.9059, -54.6732) -> (74.8201, -54.7198)
  line L85 (74.8201, -54.7198) -> (74.738, -54.7689)
  line L86 (74.738, -54.7689) -> (74.6596, -54.8206)
  line L87 (74.6596, -54.8206) -> (74.5852, -54.8747)
  line L88 (74.5852, -54.8747) -> (74.5151, -54.9312)
  line L89 (74.5151, -54.9312) -> (74.4494, -54.9901)
  line L90 (74.4494, -54.9901) -> (74.3886, -55.0514)
  line L91 (74.3886, -55.0514) -> (74.3332, -55.1151)
  line L92 (74.3332, -55.1151) -> (74.2842, -55.1816)
  line L93 (74.2842, -55.1816) -> (74.2447, -55.2518)
  line L94 (74.2447, -55.2518) -> (74.1395, -55.5251)
  line L95 (74.1395, -55.5251) -> (73.9857, -55.4706)
  line L96 (73.9857, -55.4706) -> (73.8293, -55.4242)
  line L97 (73.8293, -55.4242) -> (73.6706, -55.3861)
  line L98 (73.6706, -55.3861) -> (73.5102, -55.3565)
  line L99 (73.5102, -55.3565) -> (73.5557, -55.0672)
  line L100 (73.5557, -55.0672) -> (73.5566, -54.9866)
  line L101 (73.5566, -54.9866) -> (73.5474, -54.9046)
  line L102 (73.5474, -54.9046) -> (73.5313, -54.8217)
  line L103 (73.5313, -54.8217) -> (73.5093, -54.7382)
  line L104 (73.5093, -54.7382) -> (73.4818, -54.6544)
  line L105 (73.4818, -54.6544) -> (73.4493, -54.5703)
  line L106 (73.4493, -54.5703) -> (73.412, -54.4863)
  line L107 (73.412, -54.4863) -> (73.3699, -54.4024)
  line L108 (73.3699, -54.4024) -> (73.3234, -54.3187)
  line L109 (73.3234, -54.3187) -> (73.2724, -54.2355)
  line L110 (73.2724, -54.2355) -> (73.2171, -54.1528)
  line L111 (73.2171, -54.1528) -> (73.1575, -54.0708)
  line L112 (73.1575, -54.0708) -> (73.0722, -54.0691)
  line L113 (73.0722, -54.0691) -> (72.9869, -54.0691)
  line L114 (72.9869, -54.0691) -> (72.9016, -54.0708)
  line L115 (72.9016, -54.0708) -> (72.842, -54.1528)
  line L116 (72.842, -54.1528) -> (72.7866, -54.2355)
  line L117 (72.7866, -54.2355) -> (72.7357, -54.3187)
  line L118 (72.7357, -54.3187) -> (72.6891, -54.4024)
  line L119 (72.6891, -54.4024) -> (72.6471, -54.4863)
  line L120 (72.6471, -54.4863) -> (72.6097, -54.5703)
  line L121 (72.6097, -54.5703) -> (72.5772, -54.6544)
  line L122 (72.5772, -54.6544) -> (72.5498, -54.7382)
  line L123 (72.5498, -54.7382) -> (72.5277, -54.8217)
  line L124 (72.5277, -54.8217) -> (72.5116, -54.9046)
  line L125 (72.5116, -54.9046) -> (72.5025, -54.9866)
  line L126 (72.5025, -54.9866) -> (72.5033, -55.0672)
  line L127 (72.5033, -55.0672) -> (72.5489, -55.3565)
  line L128 (72.5489, -55.3565) -> (72.3884, -55.3861)
  line L129 (72.3884, -55.3861) -> (72.2298, -55.4242)
  line L130 (72.2298, -55.4242) -> (72.0733, -55.4706)
  line L131 (72.0733, -55.4706) -> (71.9196, -55.5251)
  line L132 (71.9196, -55.5251) -> (71.8144, -55.2518)
  line L133 (71.8144, -55.2518) -> (71.7748, -55.1816)
  line L134 (71.7748, -55.1816) -> (71.7259, -55.1151)
  line L135 (71.7259, -55.1151) -> (71.6705, -55.0514)
  line L136 (71.6705, -55.0514) -> (71.6097, -54.9901)
  line L137 (71.6097, -54.9901) -> (71.544, -54.9312)
  line L138 (71.544, -54.9312) -> (71.4738, -54.8747)
  line L139 (71.4738, -54.8747) -> (71.3994, -54.8206)
  line L140 (71.3994, -54.8206) -> (71.3211, -54.7689)
  line L141 (71.3211, -54.7689) -> (71.2389, -54.7198)
  line L142 (71.2389, -54.7198) -> (71.1531, -54.6732)
  line L143 (71.1531, -54.6732) -> (71.0639, -54.6292)
  line L144 (71.0639, -54.6292) -> (70.9713, -54.588)
  line L145 (70.9713, -54.588) -> (70.8966, -54.6292)
  line L146 (70.8966, -54.6292) -> (70.8227, -54.6719)
  line L147 (70.8227, -54.6719) -> (70.7497, -54.7159)
  line L148 (70.7497, -54.7159) -> (70.7391, -54.8168)
  line L149 (70.7391, -54.8168) -> (70.7325, -54.916)
  line L150 (70.7325, -54.916) -> (70.7299, -55.0136)
  line L151 (70.7299, -55.0136) -> (70.7314, -55.1094)
  line L152 (70.7314, -55.1094) -> (70.737, -55.203)
  line L153 (70.737, -55.203) -> (70.7467, -55.2945)
  line L154 (70.7467, -55.2945) -> (70.7605, -55.3835)
  line L155 (70.7605, -55.3835) -> (70.7787, -55.4699)
  line L156 (70.7787, -55.4699) -> (70.8013, -55.5532)
  line L157 (70.8013, -55.5532) -> (70.8288, -55.633)
  line L158 (70.8288, -55.633) -> (70.8619, -55.7086)
  line L159 (70.8619, -55.7086) -> (70.903, -55.778)
  line L160 (70.903, -55.778) -> (71.0871, -56.0058)
  line L161 (71.0871, -56.0058) -> (70.9629, -56.1117)
  line L162 (70.9629, -56.1117) -> (70.8446, -56.2239)
  line L163 (70.8446, -56.2239) -> (70.7323, -56.3423)
  line L164 (70.7323, -56.3423) -> (70.6264, -56.4665)
  line L165 (70.6264, -56.4665) -> (70.3986, -56.2823)
  line L166 (70.3986, -56.2823) -> (70.3292, -56.2413)
  line L167 (70.3292, -56.2413) -> (70.2536, -56.2082)
  line L168 (70.2536, -56.2082) -> (70.1738, -56.1807)
  line L169 (70.1738, -56.1807) -> (70.0905, -56.1581)
  line L170 (70.0905, -56.1581) -> (70.0042, -56.1399)
  line L171 (70.0042, -56.1399) -> (69.9151, -56.1261)
  line L172 (69.9151, -56.1261) -> (69.8237, -56.1164)
  line L173 (69.8237, -56.1164) -> (69.73, -56.1108)
  line L174 (69.73, -56.1108) -> (69.6343, -56.1093)
  line L175 (69.6343, -56.1093) -> (69.5367, -56.1119)
  line L176 (69.5367, -56.1119) -> (69.4374, -56.1184)
  line L177 (69.4374, -56.1184) -> (69.3366, -56.129)
  line L178 (69.3366, -56.129) -> (69.2925, -56.2021)
  line L179 (69.2925, -56.2021) -> (69.2498, -56.2759)
  line L180 (69.2498, -56.2759) -> (69.2086, -56.3506)
  line L181 (69.2086, -56.3506) -> (69.2499, -56.4433)
  line L182 (69.2499, -56.4433) -> (69.2938, -56.5325)
  line L183 (69.2938, -56.5325) -> (69.3404, -56.6183)
  line L184 (69.3404, -56.6183) -> (69.3896, -56.7005)
  line L185 (69.3896, -56.7005) -> (69.4412, -56.7788)
  line L186 (69.4412, -56.7788) -> (69.4953, -56.8532)
  line L187 (69.4953, -56.8532) -> (69.5518, -56.9233)
  line L188 (69.5518, -56.9233) -> (69.6107, -56.989)
  line L189 (69.6107, -56.989) -> (69.672, -57.0499)
  line L190 (69.672, -57.0499) -> (69.7357, -57.1052)
  line L191 (69.7357, -57.1052) -> (69.8022, -57.1542)
  line L192 (69.8022, -57.1542) -> (69.8724, -57.1937)
  line L193 (69.8724, -57.1937) -> (70.1458, -57.2989)
  line L194 (70.1458, -57.2989) -> (70.0912, -57.4527)
  line L195 (70.0912, -57.4527) -> (70.0448, -57.6091)
  line L196 (70.0448, -57.6091) -> (70.0068, -57.7678)
  line L197 (70.0068, -57.7678) -> (69.9771, -57.9283)
  line L198 (69.9771, -57.9283) -> (69.6878, -57.8827)
  line L199 (69.6878, -57.8827) -> (69.6072, -57.8819)
  line L200 (69.6072, -57.8819) -> (69.5252, -57.891)
  line L201 (69.5252, -57.891) -> (69.4423, -57.9071)
  line L202 (69.4423, -57.9071) -> (69.3588, -57.9291)
  line L203 (69.3588, -57.9291) -> (69.275, -57.9566)
  line L204 (69.275, -57.9566) -> (69.191, -57.9891)
  line L205 (69.191, -57.9891) -> (69.1069, -58.0265)
  line L206 (69.1069, -58.0265) -> (69.023, -58.0685)
  line L207 (69.023, -58.0685) -> (68.9393, -58.115)
  line L208 (68.9393, -58.115) -> (68.8561, -58.166)
  line L209 (68.8561, -58.166) -> (68.7734, -58.2214)
  line L210 (68.7734, -58.2214) -> (68.6914, -58.281)
  line L211 (68.6914, -58.281) -> (68.6897, -58.3662)
  line L212 (68.6897, -58.3662) -> (68.6897, -58.4515)
  line L213 (68.6897, -58.4515) -> (68.6914, -58.5368)
  line L214 (68.6914, -58.5368) -> (68.7734, -58.5964)
  line L215 (68.7734, -58.5964) -> (68.8561, -58.6518)
  line L216 (68.8561, -58.6518) -> (68.9393, -58.7028)
  line L217 (68.9393, -58.7028) -> (69.023, -58.7493)
  line L218 (69.023, -58.7493) -> (69.1069, -58.7913)
  line L219 (69.1069, -58.7913) -> (69.191, -58.8287)
  line L220 (69.191, -58.8287) -> (69.275, -58.8612)
  line L221 (69.275, -58.8612) -> (69.3588, -58.8887)
  line L222 (69.3588, -58.8887) -> (69.4423, -58.9107)
  line L223 (69.4423, -58.9107) -> (69.5252, -58.9268)
  line L224 (69.5252, -58.9268) -> (69.6072, -58.9359)
  line L225 (69.6072, -58.9359) -> (69.6878, -58.9351)
  line L226 (69.6878, -58.9351) -> (69.9771, -58.8895)
  line L227 (69.9771, -58.8895) -> (70.0068, -59.05)
  line L228 (70.0068, -59.05) -> (70.0448, -59.2086)
  line L229 (70.0448, -59.2086) -> (70.0912, -59.3651)
  line L230 (70.0912, -59.3651) -> (70.1458, -59.5189)
  line L231 (70.1458, -59.5189) -> (69.8724, -59.6241)
  line L232 (69.8724, -59.6241) -> (69.8022, -59.6636)
  line L233 (69.8022, -59.6636) -> (69.7357, -59.7126)
  line L234 (69.7357, -59.7126) -> (69.672, -59.7679)
  line L235 (69.672, -59.7679) -> (69.6107, -59.8288)
  line L236 (69.6107, -59.8288) -> (69.5518, -59.8945)
  line L237 (69.5518, -59.8945) -> (69.4953, -59.9646)
  line L238 (69.4953, -59.9646) -> (69.4412, -60.039)
  line L239 (69.4412, -60.039) -> (69.3896, -60.1173)
  line L240 (69.3896, -60.1173) -> (69.3404, -60.1995)
  line L241 (69.3404, -60.1995) -> (69.2938, -60.2853)
  line L242 (69.2938, -60.2853) -> (69.2499, -60.3745)
  line L243 (69.2499, -60.3745) -> (69.2086, -60.4672)
  line L244 (69.2086, -60.4672) -> (69.2498, -60.5419)
  line L245 (69.2498, -60.5419) -> (69.2925, -60.6157)
  line L246 (69.2925, -60.6157) -> (69.3366, -60.6887)
  line L247 (69.3366, -60.6887) -> (69.4374, -60.6994)
  line L248 (69.4374, -60.6994) -> (69.5367, -60.7059)
  line L249 (69.5367, -60.7059) -> (69.6343, -60.7085)
  line L250 (69.6343, -60.7085) -> (69.73, -60.707)
  line L251 (69.73, -60.707) -> (69.8237, -60.7014)
  line L252 (69.8237, -60.7014) -> (69.9151, -60.6917)
  line L253 (69.9151, -60.6917) -> (70.0042, -60.6779)
  line L254 (70.0042, -60.6779) -> (70.0905, -60.6597)
  line L255 (70.0905, -60.6597) -> (70.1738, -60.6371)
  line L256 (70.1738, -60.6371) -> (70.2536, -60.6096)
  line L257 (70.2536, -60.6096) -> (70.3292, -60.5765)
  line L258 (70.3292, -60.5765) -> (70.3986, -60.5355)
  line L259 (70.3986, -60.5355) -> (70.6264, -60.3513)
  line L260 (70.6264, -60.3513) -> (70.7323, -60.4755)
  line L261 (70.7323, -60.4755) -> (70.8446, -60.5939)
  line L262 (70.8446, -60.5939) -> (70.9629, -60.7061)
  line L263 (70.9629, -60.7061) -> (71.0871, -60.812)
  line L264 (71.0871, -60.812) -> (70.903, -61.0398)
  line L265 (70.903, -61.0398) -> (70.8619, -61.1092)
  line L266 (70.8619, -61.1092) -> (70.8288, -61.1848)
  line L267 (70.8288, -61.1848) -> (70.8013, -61.2646)
  line L268 (70.8013, -61.2646) -> (70.7787, -61.3479)
  line L269 (70.7787, -61.3479) -> (70.7605, -61.4343)
  line L270 (70.7605, -61.4343) -> (70.7467, -61.5233)
  line L271 (70.7467, -61.5233) -> (70.737, -61.6148)
  line L272 (70.737, -61.6148) -> (70.7314, -61.7084)
  line L273 (70.7314, -61.7084) -> (70.7299, -61.8042)
  line L274 (70.7299, -61.8042) -> (70.7325, -61.9017)
  line L275 (70.7325, -61.9017) -> (70.7391, -62.001)
  line L276 (70.7391, -62.001) -> (70.7497, -62.1019)
  line L277 (70.7497, -62.1019) -> (70.8227, -62.1459)
  line L278 (70.8227, -62.1459) -> (70.8966, -62.1886)
  line L279 (70.8966, -62.1886) -> (70.9713, -62.2298)
  line L280 (70.9713, -62.2298) -> (71.0639, -62.1886)
  line L281 (71.0639, -62.1886) -> (71.1531, -62.1446)
  line L282 (71.1531, -62.1446) -> (71.2389, -62.098)
  line L283 (71.2389, -62.098) -> (71.3211, -62.0489)
  line L284 (71.3211, -62.0489) -> (71.3994, -61.9972)
  line L285 (71.3994, -61.9972) -> (71.4738, -61.9431)
  line L286 (71.4738, -61.9431) -> (71.544, -61.8866)
  line L287 (71.544, -61.8866) -> (71.6097, -61.8277)
  line L288 (71.6097, -61.8277) -> (71.6705, -61.7664)
  line L289 (71.6705, -61.7664) -> (71.7259, -61.7027)
  line L290 (71.7259, -61.7027) -> (71.7748, -61.6362)
  line L291 (71.7748, -61.6362) -> (71.8144, -61.566)
  line L292 (71.8144, -61.566) -> (71.9196, -61.2927)
  line L293 (71.9196, -61.2927) -> (72.0733, -61.3472)
  line L294 (72.0733, -61.3472) -> (72.2298, -61.3936)
  line L295 (72.2298, -61.3936) -> (72.3884, -61.4317)
  line L296 (72.3884, -61.4317) -> (72.5489, -61.4613)
  line L297 (72.5489, -61.4613) -> (72.5033, -61.7506)
  line L298 (72.5033, -61.7506) -> (72.5025, -61.8312)
  line L299 (72.5025, -61.8312) -> (72.5116, -61.9132)
  line L300 (72.5116, -61.9132) -> (72.5277, -61.9961)
  line L301 (72.5277, -61.9961) -> (72.5498, -62.0796)
  line L302 (72.5498, -62.0796) -> (72.5772, -62.1634)
  line L303 (72.5772, -62.1634) -> (72.6097, -62.2475)
  line L304 (72.6097, -62.2475) -> (72.6471, -62.3315)
  line L305 (72.6471, -62.3315) -> (72.6891, -62.4154)
  line L306 (72.6891, -62.4154) -> (72.7357, -62.4991)
  line L307 (72.7357, -62.4991) -> (72.7866, -62.5823)
  line L308 (72.7866, -62.5823) -> (72.842, -62.665)
  line L309 (72.842, -62.665) -> (72.9016, -62.747)
  line L310 (72.9016, -62.747) -> (72.9869, -62.7487)
  line L311 (72.9869, -62.7487) -> (73.0722, -62.7487)
  line L312 (73.0722, -62.7487) -> (73.1575, -62.747)
  line L313 (73.1575, -62.747) -> (73.2171, -62.665)
  line L314 (73.2171, -62.665) -> (73.2724, -62.5823)
  line L315 (73.2724, -62.5823) -> (73.3234, -62.4991)
  line L316 (73.3234, -62.4991) -> (73.3699, -62.4154)
  line L317 (73.3699, -62.4154) -> (73.412, -62.3315)
  line L318 (73.412, -62.3315) -> (73.4493, -62.2475)
  line L319 (73.4493, -62.2475) -> (73.4818, -62.1634)
  line L320 (73.4818, -62.1634) -> (73.5093, -62.0796)
  line L321 (73.5093, -62.0796) -> (73.5313, -61.9961)
  line L322 (73.5313, -61.9961) -> (73.5474, -61.9132)
  line L323 (73.5474, -61.9132) -> (73.5566, -61.8312)
  line L324 (73.5566, -61.8312) -> (73.5557, -61.7506)
  line L325 (73.5557, -61.7506) -> (73.5102, -61.4613)
  line L326 (73.5102, -61.4613) -> (73.6706, -61.4317)
  line L327 (73.6706, -61.4317) -> (73.8293, -61.3936)
  line L328 (73.8293, -61.3936) -> (73.9857, -61.3472)
  line L329 (73.9857, -61.3472) -> (74.1395, -61.2927)
  line L330 (74.1395, -61.2927) -> (74.2447, -61.566)
  line L331 (74.2447, -61.566) -> (74.2842, -61.6362)
  line L332 (74.2842, -61.6362) -> (74.3332, -61.7027)
  line L333 (74.3332, -61.7027) -> (74.3886, -61.7664)
  line L334 (74.3886, -61.7664) -> (74.4494, -61.8277)
  line L335 (74.4494, -61.8277) -> (74.5151, -61.8866)
  line L336 (74.5151, -61.8866) -> (74.5852, -61.9431)
  line L337 (74.5852, -61.9431) -> (74.6596, -61.9972)
  line L338 (74.6596, -61.9972) -> (74.738, -62.0489)
  line L339 (74.738, -62.0489) -> (74.8201, -62.098)
  line L340 (74.8201, -62.098) -> (74.9059, -62.1446)
  line L341 (74.9059, -62.1446) -> (74.9952, -62.1886)
  line L342 (74.9952, -62.1886) -> (75.0878, -62.2298)
  line L343 (75.0878, -62.2298) -> (75.1625, -62.1886)
  line L344 (75.1625, -62.1886) -> (75.2364, -62.1459)
  line L345 (75.2364, -62.1459) -> (75.3094, -62.1019)
  line L346 (75.3094, -62.1019) -> (75.32, -62.001)
  line L347 (75.32, -62.001) -> (75.3266, -61.9017)
  line L348 (75.3266, -61.9017) -> (75.3291, -61.8042)
  line L349 (75.3291, -61.8042) -> (75.3276, -61.7084)
  line L350 (75.3276, -61.7084) -> (75.322, -61.6148)
  line L351 (75.322, -61.6148) -> (75.3124, -61.5233)
  line L352 (75.3124, -61.5233) -> (75.2985, -61.4343)
  line L353 (75.2985, -61.4343) -> (75.2804, -61.3479)
  line L354 (75.2804, -61.3479) -> (75.2577, -61.2646)
  line L355 (75.2577, -61.2646) -> (75.2302, -61.1848)
  line L356 (75.2302, -61.1848) -> (75.1971, -61.1092)
  line L357 (75.1971, -61.1092) -> (75.1561, -61.0398)
  line L358 (75.1561, -61.0398) -> (74.972, -60.812)